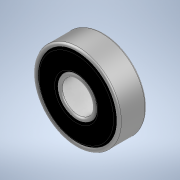
# Autodesk Inventor part: Bearing
Saved by Autodesk Inventor 2021 (Build 250183000, 183)
## iProperties
Created: 2021-06-08
Part Number: Bearing
Material: Generic
Document SubType Name: Modeling
Designer: zmac845
Density: 1 g/cm^3
Appearance: Default
Author: zmac845
Autodesk Inventor part; units mm, degrees
ref_plane "YZ Plane" through (0, 0, 0) normal (1, 0, 0) x (0, 1, 0)
ref_plane "XZ Plane" through (0, 0, 0) normal (0, 1, 0) x (-1, 0, 0)
ref_plane "XY Plane" through (0, 0, 0) normal (0, 0, 1) x (1, 0, 0)
sketch "Sketch1" plane through (0, 0, 0) normal (0, 0, 1) x (1, 0, 0)
  circle A0 centre (0, 0) radius 4
  circle A1 centre (0, 0) radius 11
  circle A2 centre (0, 0) radius 5
  circle A3 centre (0, 0) radius 10
  dimension "d0" = 8
  dimension "d1" = 22
  dimension "d2" = 10
  dimension "d3" = 20
  constraints: 4 centre point, 4 coincident
  measures "d0" diameter of A0
  measures "d1" diameter of A1
  measures "d2" diameter of A2
  measures "d3" diameter of A3
extrude "Extrusion1" add sketch "Sketch1" along normal blind 7 contours A2
fillet "Fillet1" radius 0.5 4 edges at (-5, 0, 7) (-4, 0, 7) (-5, 0, 0) (-4, 0, 0)
extrude "Extrusion2" add sketch "Sketch1" along normal blind 7 contours A1
fillet "Fillet3" radius 0.5 4 edges at (-10, 0, 7) (-11, 0, 7) (-11, 0, 0) (-10, 0, 0)
extrude "Extrusion3" add sketch "Sketch1" along normal blind 7 contours A3
fillet "Fillet4" radius 0.5 4 edges at (-10, 0, 7) (-5, 0, 7) (-10, 0, 0) (-5, 0, 0)
body "Solid1"
